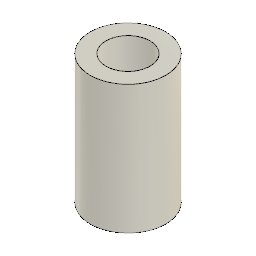
Radiační kryt SESTAVA v9 (Autodesk Fusion 360 archive; units mm, degrees)
design "Sloupek(radiackniKryt)"
Autodesk Fusion 360 part; units mm, degrees
note: some values were not read from the file. Set by a fixed rule: which sketch regions a step uses.
sketch "Sketch1" plane through (0, 0, 0) normal (0, 0, 1) x (1, 0, 0)
  circle A0 centre (0, 0) radius 3.6
  circle A1 centre (0, 0) radius 2.1
  dimension "d1" = 7.2
  dimension "d2" = 4.2
  constraint coincident A0.centre A1.centre
  constraint concentric A0 A1
  measures "d1" diameter of A0
  measures "d2" diameter of A1
extrude "Extrude1" add sketch "Sketch1" along normal blind 12.3

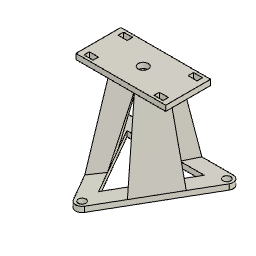
design "radiační kryt_uchyt"
Autodesk Fusion 360 part; units mm, degrees
sketch "Sketch1" plane through (0, 0, 0) normal (0, 0, 1) x (1, 0, 0)
  line L0 (0, 0) -> (0, 17.037)
  line L1 (0, 17.037) -> (29.509, 17.037)
  line L2 (0, 17.037) -> (-29.509, 17.037)
  line L3 (29.509, 17.037) -> (0, -34.0741)
  line L4 (29.509, 17.037) -> (88.527, 17.037) construction
  line L5 (-29.509, 17.037) -> (0, -34.0741)
  circle A0 centre (-29.509, 17.037) radius 2.1
  circle A1 centre (-29.509, 17.037) radius 3.6
  circle A2 centre (0, -34.074) radius 3.6
  circle A3 centre (0, -34.074) radius 2.1
  circle A4 centre (29.509, 17.037) radius 3.6
  circle A5 centre (29.509, 17.037) radius 2.1
  line L6 (-29.509, 20.637) -> (29.509, 20.637)
  line L7 (-29.509, 13.437) -> (29.509, 13.437)
  line L8 (3.1177, -32.274) -> (-26.3913, 18.837)
  line L9 (-3.1177, -35.874) -> (-32.6267, 15.237)
  line L10 (26.3913, 18.837) -> (-3.1177, -32.274)
  line L11 (32.6267, 15.237) -> (3.1177, -35.874)
  line L12 (-29.509, 12.437) -> (29.509, 12.437)
  line L13 (3.9837, -31.774) -> (-25.5253, 19.337)
  line L14 (25.5253, 19.337) -> (-3.9837, -31.774)
  dimension "d1" = 17.037
  dimension "d2" = 29.509
  dimension "d3" = 29.509
  dimension "d4" = 120
  dimension "d5" = 59.018
  dimension "d6" = 4.2
  dimension "d7" = 7.2
  dimension "d9" = 360
  dimension "d11" = 360
  dimension "d12" = 1
  dimension "d14" = 360
  constraint coincident L0.start origin
  constraint vertical L0
  constraint perpendicular L0 L1
  constraint perpendicular L0 L2
  constraint horizontal L4
  constraint coincident L2.end L5.start
  constraint concentric A0 A1
  constraint coincident A1 L6.start
  constraint coincident A4 L6.end
  constraint tangent A4 L6
  constraint coincident A1 L7.start
  constraint coincident A4 L7.end
  constraint tangent A4 L7
  constraint parallel L6 L7
  measures "d1" distance of L0.start L0.end
  measures "d2" distance of L0.end L1.end
  measures "d3" distance of L0.end L2.end
  measures "d4" angle of L3 L4
  measures "d5" distance of L1.end L3.end
  measures "d6" diameter of A0
  measures "d7" diameter of A1
extrude "Extrude1" add sketch "Sketch1" along normal blind 3 contours L0 L7 L12 L13 | L0 L7 L12 L14 | L0 L2 L7 L13 | L0 L1 L7 L14 | L8 L12 L13 L14 | L7 L8 L12 L13 | L7 L10 L12 L14 | L10 L12 L13 L14 | L1 L2 A1 A4 L6 L8 L10 | L2 L7 L8 L13 | L1 L7 L10 L14 | L5 L7 L8 L12 | L5 L8 L12 L14 | L8 L10 L13 L14 | L3 L10 L12 L13 | L3 L7 L10 L12 | L2 L5 A1 L7 L8 | L1 L3 A4 L7 L10 | L5 L8 L10 L14 | L5 A1 A2 L7 L9 L10 | L3 L8 L10 L13 | L3 A2 A4 L7 L8 L11 | L1 A4 L10 | L2 A1 L8 | L5 A1 L7 | L3 A4 L7 | L3 L5 A2 L8 L10 | L1 L3 A4 A5 | L1 L3 A4 A5 | L2 L5 A0 A1 | L2 L5 A0 A1 | L3 A2 L8 | L5 A2 L10 | L3 L5 A2 A3 | L3 L5 A2 A3 makes body 1
ref_plane "WorkPlane1" through (0, -8.5185, 48) normal (0, 0, 1) x (1, 0, 0)
sketch "Sketch2" plane through (0, 0, 48) normal (0, 0, 1) x (1, 0, 0)
  line L0 (0, 0) -> (25, 0)
  line L1 (25, 0) -> (25, 12.5)
  line L2 (25, 12.5) -> (0, 12.5)
  line L3 (0, 12.5) -> (0, 0)
  line L4 (25, 12.5) -> (-25, 12.5)
  line L5 (-25, 12.5) -> (-25, -12.5)
  line L6 (-25, -12.5) -> (25, -12.5)
  line L7 (25, -12.5) -> (25, 12.5)
  line L8 (0, 12.5) -> (7, 12.5)
  line L9 (7, 12.5) -> (-7, 12.5)
  line L10 (0, 0) -> (0, 1)
  line L11 (0, 1) -> (1, 1)
  line L12 (1, 1) -> (-1, 1)
  line L13 (-7, 12.5) -> (-1, 1)
  line L14 (1, 1) -> (7, 12.5)
  line L15 (-7, 12.5) -> (7, 12.5)
  line L16 (-7.3253, -12.3122) -> (-0.366, -1.366)
  line L17 (-7.3253, -12.3122) -> (-14.3253, -0.1878)
  line L18 (-1.366, 0.366) -> (-14.3253, -0.1878)
  line L19 (-1.366, 0.366) -> (-0.366, -1.366)
  line L20 (14.3253, -0.1878) -> (1.366, 0.366)
  line L21 (14.3253, -0.1878) -> (7.3253, -12.3122)
  line L22 (0.366, -1.366) -> (7.3253, -12.3122)
  line L23 (0.366, -1.366) -> (1.366, 0.366)
  line L24 (0, 0) -> (-17, 0)
  line L25 (-17, 0) -> (-17, -8)
  line L26 (-17, -8) -> (0, -8)
  line L27 (0, -8) -> (0, 0)
  line L28 (-17, -8) -> (17, -8)
  line L29 (17, -8) -> (17, 8)
  line L30 (17, 8) -> (-17, 8)
  line L31 (-17, 8) -> (-17, -8)
  line L32 (17, 8) -> (22, 8)
  line L33 (22, 8) -> (22, 11)
  line L34 (22, 11) -> (17, 11)
  line L35 (17, 11) -> (17, 8)
  line L36 (-17, 8) -> (-22, 8)
  line L37 (-17, 11) -> (-17, 8)
  line L38 (-22, 11) -> (-17, 11)
  line L39 (-22, 8) -> (-22, 11)
  line L40 (-22, -11) -> (-17, -11)
  line L41 (-22, -8) -> (-22, -11)
  line L42 (-17, -8) -> (-22, -8)
  line L43 (-17, -11) -> (-17, -8)
  line L44 (17, -11) -> (17, -8)
  line L45 (22, -11) -> (17, -11)
  line L46 (17, -8) -> (22, -8)
  line L47 (22, -8) -> (22, -11)
  point P0 (-17, -8)
  dimension "d18" = 25
  dimension "d19" = 12.5
  dimension "d20" = 50
  dimension "d21" = 25
  dimension "d22" = 7
  dimension "d23" = 14
  dimension "d32" = 1
  dimension "d33" = 1
  dimension "d34" = 2
  dimension "d36" = 360
  dimension "d37" = 17
  dimension "d38" = 8
  dimension "d39" = 34
  dimension "d40" = 16
  dimension "d41" = 5
  dimension "d42" = 3
  constraint horizontal L0
  constraint vertical L1
  constraint horizontal L2
  constraint vertical L3
  constraint coincident L0.start L3.end
  constraint horizontal L4
  constraint vertical L5
  constraint horizontal L6
  constraint vertical L7
  constraint perpendicular L3 L8
  constraint perpendicular L3 L9
  constraint parallel L3 L10
  constraint perpendicular L3 L11
  constraint perpendicular L10 L12
  constraint horizontal L24
  constraint vertical L25
  constraint horizontal L26
  constraint vertical L27
  constraint horizontal L28
  constraint vertical L29
  constraint horizontal L30
  constraint vertical L31
  constraint horizontal L32
  constraint vertical L33
  constraint horizontal L34
  constraint vertical L35
  constraint symmetric L3 L29.end L30.end
  constraint symmetric L3 L32.end L36.end
  constraint symmetric L3 L33.end L38.start
  constraint symmetric L3 L34.end L37.start
  constraint symmetric L24 L29.end L28.end
  constraint symmetric L24 L30.end P0
  constraint symmetric L24 L32.end L46.end
  constraint symmetric L24 L33.end L45.start
  constraint symmetric L24 L34.end L44.start
  constraint symmetric L24 L36.end L41.start
  constraint symmetric L24 L37.start L40.end
  constraint symmetric L24 L38.start L40.start
  measures "d18" distance of L0.start L0.end
  measures "d19" distance of L0.start L2.end
  measures "d20" distance of L1.end L4.end
  measures "d21" distance of L1.end L6.end
  measures "d22" distance of L2.end L8.end
  measures "d23" distance of L8.end L9.end
  measures "d32" distance of L0.start L10.end
  measures "d33" distance of L10.end L11.end
  measures "d34" distance of L11.end L12.end
  measures "d37" distance of L0.start L24.end
  measures "d38" distance of L0.start L26.end
  measures "d39" distance of P0 L28.end
  measures "d40" distance of P0 L30.end
  measures "d41" distance of L29.end L32.end
  measures "d42" distance of L29.end L34.end
sketch "Sketch3" plane through (0, 0, 3) normal (0, 0, 1) x (-1, 0, 0)
  circle A0 centre (29.509, -17.037) radius 2.1
  line L0 (0, 24.874) -> (21.5416, -12.437)
  line L1 (21.5416, -12.437) -> (-21.5415, -12.437)
  line L2 (-21.5415, -12.437) -> (0, 24.874)
  circle A1 centre (0, 34.074) radius 2.1
  circle A2 centre (-29.509, -17.037) radius 2.1
  arc A3 (29.509, -20.637) -> (32.6267, -15.237) centre (29.509, -17.037) ccw
  line L3 (32.6267, -15.237) -> (3.1177, 35.874)
  arc A4 (3.1177, 35.874) -> (-3.1177, 35.874) centre (0, 34.074) ccw
  line L4 (-3.1177, 35.874) -> (-32.6267, -15.237)
  arc A5 (-32.6267, -15.237) -> (-29.509, -20.637) centre (-29.509, -17.037) ccw
  line L5 (-29.509, -20.637) -> (29.509, -20.637)
  line L6 (0, -12.437) -> (-8, -12.437)
  line L7 (-8, -12.437) -> (8, -12.437)
  line L8 (0, -20.637) -> (-12, -20.637)
  line L9 (-12, -20.637) -> (12, -20.637)
  line L10 (12, -20.637) -> (8, -12.437)
  line L11 (-12, -20.637) -> (-8, -12.437)
  line L12 (11.8722, 20.7108) -> (6.7708, 13.1467)
  line L13 (23.8722, -0.0738) -> (11.8722, 20.7108)
  line L14 (14.7708, -0.7097) -> (6.7708, 13.1467)
  line L15 (23.8722, -0.0738) -> (14.7708, -0.7097)
  line L16 (-23.8722, -0.0738) -> (-14.7708, -0.7097)
  line L17 (-11.8722, 20.7108) -> (-23.8722, -0.0738)
  line L18 (-6.7708, 13.1467) -> (-14.7708, -0.7097)
  line L19 (-11.8722, 20.7108) -> (-6.7708, 13.1467)
  dimension "d26" = 8
  dimension "d27" = 16
  dimension "d28" = 12
  dimension "d29" = 24
  dimension "d31" = 360
  constraint midpoint L1 L6.start
  constraint parallel L1 L6
  constraint parallel L1 L7
  constraint midpoint L5 L8.start
  constraint parallel L5 L8
  constraint parallel L5 L9
  measures "d26" distance of L6.start L6.end
  measures "d27" distance of L6.end L7.end
  measures "d28" distance of L8.start L8.end
  measures "d29" distance of L8.end L9.end
loft "Loft2" add profiles "Sketch3", "Sketch2" section 1 contours L1 L5 L6 L7 L8 L9 L10 L11 section 2 contours L3 L12 L13 L30 | L3 L11 L12 L14 L30 | L3 L4 L9 L13 L15 L30 | L2 L3 L4 L8 L9 L14 L15 L30 separate body makes body 2
loft "Loft3" add profiles "Sketch3", "Sketch2" section 1 contours L2 L4 L16 L17 L18 L19 section 2 contours L0 L20 L23 | L0 L20 L21 L22 L23 L28 | L21 L22 L28 separate body makes body 3
loft "Loft4" add profiles "Sketch3", "Sketch2" section 1 contours L0 L3 L12 L13 L14 L15 section 2 contours L18 L19 L24 | L16 L17 L18 L19 L24 L26 L28 | L16 L17 L26 L28 separate body makes body 4
extrude "Extrude2" add sketch "Sketch2" along normal blind 3 separate body makes body 5
sketch "Sketch4" plane through (0, 0, 48) normal (0, 0, -1) x (1, 0, 0)
  line L0 (-17, 11) -> (-17, 8)
  line L1 (-17, 8) -> (-22, 8)
  line L2 (-22, 8) -> (-22, 11)
  line L3 (-22, 11) -> (-17, 11)
  line L4 (17, -11) -> (17, -8)
  line L5 (17, -8) -> (22, -8)
  line L6 (22, -8) -> (22, -11)
  line L7 (22, -11) -> (17, -11)
  line L8 (-22, -8) -> (-17, -8)
  line L9 (-17, -8) -> (-17, -11)
  line L10 (-17, -11) -> (-22, -11)
  line L11 (-22, -11) -> (-22, -8)
  line L12 (22, 8) -> (17, 8)
  line L13 (17, 8) -> (17, 11)
  line L14 (17, 11) -> (22, 11)
  line L15 (22, 11) -> (22, 8)
  line L16 (-25, 12.5) -> (-25, -12.5)
  line L17 (-25, -12.5) -> (25, -12.5)
  line L18 (25, -12.5) -> (25, 12.5)
  line L19 (25, 12.5) -> (-25, 12.5)
  circle A0 centre (0, 0) radius 2.75
  dimension "d45" = 5.5
  constraint coincident A0.centre origin
  measures "d45" diameter of A0
extrude "Extrude3" cut sketch "Sketch4" along normal blind 20 and the other way blind 6 contours A0 bodies 2 3 4 5
equation "d2 = ( 59.018 / 2 ) * 1 mm"
equation "d3 = ( 59.018 / 2 ) * 1 mm"
equation "d19 = ( 25 / 2 ) * 1 mm"
equation "d22 = ( 14 / 2 ) * 1 mm"
equation "d37 = ( 34 / 2 ) * 1 mm"
equation "d38 = ( 16 / 2 ) * 1 mm"
